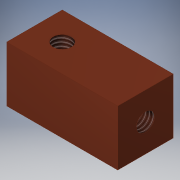
# Autodesk Inventor part: alublock
Saved by Autodesk Inventor 2018.3 (Build 223285000, 285)
## iProperties
Created: 2021-01-25
Part Number: alublock
Material: Kupfer
Document SubType Name: Modeling
Designer: stege
Density: 8.94 g/cm^3
Appearance: Kupfer - satiniert
Author: stege
Autodesk Inventor part; units mm, degrees
ref_plane "YZ Plane" through (0, 0, 0) normal (1, 0, 0) x (0, 1, 0)
ref_plane "XZ Plane" through (0, 0, 0) normal (0, 1, 0) x (-1, 0, 0)
ref_plane "XY Plane" through (0, 0, 0) normal (0, 0, 1) x (1, 0, 0)
sketch "Skizze1" plane through (0, 0, 0) normal (0, 1, 0) x (-1, 0, 0)
  line L0 (15, -7.5) -> (-15, -7.5)
  line L1 (-15, -7.5) -> (-15, 7.5)
  line L2 (-15, 7.5) -> (15, 7.5)
  line L3 (15, 7.5) -> (15, -7.5)
  line L4 (15, -7.5) -> (-15, 7.5) construction
  line L5 (-15, -7.5) -> (15, 7.5) construction
  point P0 (0, 0)
  dimension "d0" = 15
  dimension "d1" = 30
  constraints: 12 end point, 2 midpoint, 2 parallel, 1 horizontal, 1 perpendicular
  measures "d0" distance of L0.end L1.end
  measures "d1" distance of L0.start L0.end
extrude "Extrusion1" add sketch "Skizze1" along normal blind 15
sketch "Skizze2" plane through (15, 0, 7.5) normal (1, 0, 0) x (0, 0, -1)
  circle A0 centre (7.5, 7.5) radius 4
  line L0 (0, 0) -> (0, 15) projected
  point P0 (7.5, 0)
  dimension "d4" = 7.5
  dimension "d5" = 8
  dimension "d47" = 7.5
  constraints: 1 centre point
  measures "d4" distance of point (7.5, 0) A0.centre
  measures "d5" diameter of A0
  measures "d47" distance from line of L0 A0.centre
hole "Bohrung1" at (15, 7.5, 0) direction (-1, 0, 0) diameter 4.917 depth 20 tip angle 118 thread size "M6x1" class "6H" standard "ISO Metric profile"
sketch "Skizze4" plane through (-15, 0, 7.5) normal (0, 0, 1) x (1, 0, 0)
  circle A0 centre (7.5, 7.5) radius 2.1663
  line L0 (30, 0) -> (0, 0) projected
  line L1 (0, 0) -> (0, 15) projected
  circle A1 centre (22, 15) radius 3.1386
  line L2 (30, 0) -> (30, 15) projected
  point P0 (15, 0)
  dimension "d27" = 7.5
  dimension "d28" = 7.5
  dimension "d29" = 15
  dimension "d30" = 8
  constraints: 2 centre point
  measures "d27" distance from line of L0 A0.centre
  measures "d28" distance from line of L1 A0.centre
  measures "d29" distance from line of L0 A1.centre
  measures "d30" distance from line of L2 A1.centre
hole "Bohrung3" at (-7.5, 7.5, 7.5) direction (0, 0, -1) diameter 4.917 depth 15 tip angle 118 thread size "M6x1" class "6H" standard "ISO Metric profile"
